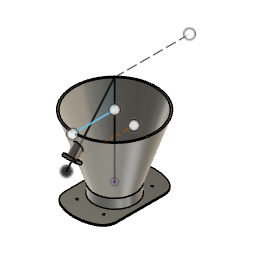
DroneVibrationSensorDeploymentCone-Remake v3 (Autodesk Fusion 360 design; units mm, degrees)
Autodesk Fusion 360 part; units mm, degrees
note: some values were not read from the file. Chosen so that the rebuilt part matches the saved one: which bodies a step acts on; which face or edge a step refers to; which pieces of a blend or face edit are solid.
sketch "Sketch1" plane through (0, 0, 0) normal (0, 1, 0) x (1, 0, 0)
  line L0 (0, 0) -> (32.2, 0)
  line L1 (0, 0) -> (0, -100)
  line L2 (0, -100) -> (65.7, -100)
  line L3 (65.7, -100) -> (32.2, 0)
  dimension "d1" = 32.2
  dimension "d2" = 100
  dimension "d3" = 65.7
  constraint coincident L0.start L1.start
  constraint horizontal L0
  constraint perpendicular L0 L1
  constraint perpendicular L1 L2
  measures "d1" distance of L0.start L0.end
  measures "d2" distance of L0.start L1.end
  measures "d3" distance of L1.end L2.end
revolve "Revolve1" add sketch "Sketch1" angle 360 about axis through (0, 0, 0) along (0, 0, 1) makes body 1
shell "Shell1" thickness 2.5 removed faces 1 at (2.2714, -9.9517, 100) on bodies 1
sketch "Sketch2" plane through (0, 0, 0) normal (0, 0, -1) x (1, 0, 0)
  circle A0 centre (0, 0) radius 32.2
  line L0 (-21, -21) -> (21, -21)
  line L1 (21, -21) -> (21, 21)
  line L2 (21, 21) -> (-21, 21)
  line L3 (-21, 21) -> (-21, -21)
  circle A1 centre (0, 0) radius 32.5
  dimension "d6" = 42
  dimension "d7" = 42
  constraint horizontal L0
  constraint vertical L1
  constraint horizontal L2
  constraint vertical L3
  constraint coincident A0.centre A1.centre
  measures "d6" distance of L0.start L0.end
  measures "d7" distance of L0.start L2.end
extrude "Extrude1" add sketch "Sketch2" along normal blind 22.5 contours A0 | L0 L1 L2 L3 | A1 bodies 1
extrude "Extrude2" cut sketch "Sketch2" against normal blind 10 contours L0 L1 L2 L3 bodies 1
extrude "Extrude3" cut sketch "Sketch2" along normal blind 16 contours L0 L1 L2 L3 bodies 1
sketch "Sketch5" plane through (0, 0, -16) normal (0, 0, 1) x (-1, 0, 0)
  line L0 (21, -21) -> (21, 21)
  line L1 (21, 21) -> (-21, 21)
  line L2 (-21, 21) -> (-21, -21)
  line L3 (-21, -21) -> (21, -21)
  circle A0 centre (17.5, -17.5) radius 1.5
  circle A1 centre (-17.5, -17.5) radius 1.5
  circle A2 centre (17.5, 17.5) radius 1.5
  circle A3 centre (-17.5, 17.5) radius 1.5
  line L4 (21, 21) -> (28.894, 21) construction
  line L5 (18.4952, 13.5139) -> (3.4952, 13.5139)
  line L6 (3.4952, 13.5139) -> (3.4952, -1.4861)
  line L7 (3.4952, -1.4861) -> (18.4952, -1.4861)
  line L8 (18.4952, -1.4861) -> (18.4952, 13.5139)
  dimension "d17" = 15
  dimension "d18" = 15
  constraint horizontal L4
  constraint coincident L0.end L1.start
  constraint horizontal L5
  constraint vertical L6
  constraint horizontal L7
  constraint vertical L8
  measures "d17" distance of L5.start L5.end
  measures "d18" distance of L5.start L7.end
extrude "Extrude4" cut sketch "Sketch5" against normal blind 1 contours A0 | A1 | A2 | A3 | L5 L6 L7 L8 bodies 1
extrude "Extrude5" cut 1 faces at (-1.1612, -8.4698, -22.5) along direction (0, 0, 1) blind 5.5 on bodies 1 bodies 1
sketch "Sketch6" plane through (0, 0, -17) normal (0, 0, -1) x (1, 0, 0)
  circle A0 centre (-17.5, -17.5) radius 1.5
  line L0 (-18.4952, 13.5139) -> (-3.4952, 13.5139)
  line L1 (-3.4952, 13.5139) -> (-3.4952, -1.4861)
  line L2 (-3.4952, -1.4861) -> (-18.4952, -1.4861)
  line L3 (-18.4952, -1.4861) -> (-18.4952, 13.5139)
  circle A1 centre (17.5, -17.5) radius 1.5
  circle A2 centre (-17.5, 17.5) radius 1.5
  circle A3 centre (17.5, 17.5) radius 1.5
  circle A4 centre (0, 0) radius 32.5
  line L4 (-18.4952, 13.5139) -> (-3.4952, 13.5139)
  line L5 (-3.4952, 13.5139) -> (-3.4952, -1.4861)
  line L6 (-3.4952, -1.4861) -> (-18.4952, -1.4861)
  line L7 (-18.4952, -1.4861) -> (-18.4952, 13.5139)
  circle A5 centre (-17.5, 17.5) radius 1.5
  circle A6 centre (17.5, 17.5) radius 1.5
  circle A7 centre (17.5, -17.5) radius 1.5
  circle A8 centre (-17.5, -17.5) radius 1.5
  circle A9 centre (0, 0) radius 65
  line L8 (0, 0) -> (44.414, 0) construction
  line L9 (0, 0) -> (44.414, 0) construction
  line L10 (0, 0) -> (44.414, 0) construction
  line L11 (0, 0) -> (44.414, 0) construction
  circle A10 centre (21.2606, -38.9947) radius 1.5
  circle A11 centre (-21.2606, -38.9947) radius 1.5
  circle A12 centre (-21.2606, 38.9947) radius 1.5
  circle A13 centre (21.2606, 38.9947) radius 1.5
  line L12 (0, 0) -> (65, 0)
  line L13 (0, 0) -> (0, 65)
  line L14 (0, -65) -> (0, 0)
  line L15 (0, 0) -> (-65, 0)
  dimension "d23" = 130
  dimension "d32" = 3
  dimension "d33" = 3
  dimension "d34" = 3
  dimension "d35" = 3
  constraint horizontal L4
  constraint vertical L5
  constraint horizontal L6
  constraint vertical L7
  constraint coincident L1.end L2.start
  constraint coincident L0.start L3.end
  constraint concentric A2 A5
  constraint concentric A3 A6
  constraint concentric A1 A7
  constraint concentric A0 A8
  constraint coincident A4.centre A9.centre
  constraint horizontal L8
  constraint horizontal L9
  constraint horizontal L10
  constraint horizontal L11
  constraint coincident A9 L12.end
  constraint parallel L9 L12
  constraint coincident A9 L13.end
  constraint perpendicular L10 L13
  constraint coincident A9 L14.start
  constraint perpendicular L12 L14
  constraint coincident A9 L15.end
  constraint perpendicular L5 L15
  measures "d23" diameter of A9
  measures "d32" diameter of A10
  measures "d33" diameter of A11
  measures "d34" diameter of A12
  measures "d35" diameter of A13
extrude "Extrude6" add sketch "Sketch6" against normal blind 2 contours A4 A9 L13 L15 | A4 A9 L14 L15 | A4 A9 L12 L13 | A4 A9 L12 L14 bodies 1
sketch "Sketch7" plane through (0, 0, -17) normal (0, 0, -1) x (1, 0, 0)
  circle A0 centre (0, 0) radius 65
  circle A1 centre (21.2606, 38.9947) radius 1.5
  circle A2 centre (-21.2606, 38.9947) radius 1.5
  circle A3 centre (21.2606, -38.9947) radius 1.5
  circle A4 centre (-21.2606, -38.9947) radius 1.5
  circle A5 centre (-17.5, -17.5) radius 1.5
  line L0 (-18.4952, 13.5139) -> (-3.4952, 13.5139)
  line L1 (-3.4952, 13.5139) -> (-3.4952, -1.4861)
  line L2 (-3.4952, -1.4861) -> (-18.4952, -1.4861)
  line L3 (-18.4952, -1.4861) -> (-18.4952, 13.5139)
  circle A6 centre (17.5, -17.5) radius 1.5
  circle A7 centre (-17.5, 17.5) radius 1.5
  circle A8 centre (17.5, 17.5) radius 1.5
  line L4 (0, 0) -> (41.407, 0)
  line L5 (0, 0) -> (-41.407, 0)
  line L6 (-41.407, 0) -> (-41.407, 50.1045)
  line L7 (-41.407, 0) -> (-41.407, -50.1045)
  line L8 (41.407, 0) -> (41.407, 50.1045)
  line L9 (41.407, 50.1045) -> (41.407, -50.1045)
  dimension "d38" = 41.407
  dimension "d39" = 41.407
  constraint coincident A0.centre L4.start
  constraint horizontal L4
  constraint parallel L4 L5
  constraint coincident A0 L6.end
  constraint perpendicular L5 L6
  constraint coincident A0 L7.end
  constraint perpendicular L5 L7
  constraint coincident A0 L8.end
  constraint perpendicular L4 L8
  constraint coincident A0 L9.end
  constraint perpendicular L4 L9
  measures "d38" distance of A0.centre L4.end
  measures "d39" distance of A0.centre L5.end
extrude "Extrude7" cut sketch "Sketch7" against normal blind 2 contours A0 L8 L9 | A0 L6 L7 bodies 1
fillet "Fillet1" radius 22.5 4 edges at (-41.407, -50.1045, -16) (41.407, -50.1045, -16) (41.407, 50.1045, -16) (-41.407, 50.1045, -16) on bodies 1
sketch "Sketch8" plane through (0, 0, 0) normal (0, 0, 1) x (1, 0, 0)
  line L0 (7.25, -37.9) -> (-7.25, -37.9)
  line L1 (7.25, -37.9) -> (-7.25, -37.9)
  line L2 (-7.25, -37.9) -> (-7.25, -52)
  line L3 (-7.25, -52) -> (7.25, -52)
  line L4 (7.25, -52) -> (7.25, -37.9)
  line L5 (7.25, -37.9) -> (9.25, -37.9) construction
  line L6 (-7.25, -52) -> (-5.25, -52) construction
  line L7 (8.6642, -36.4858) -> (-8.6642, -36.4858)
  line L8 (-8.6642, -36.4858) -> (-8.6642, -53.4142)
  line L9 (-8.6642, -53.4142) -> (8.6642, -53.4142)
  line L10 (8.6642, -53.4142) -> (8.6642, -36.4858)
  dimension "d47" = 14.5
  constraint horizontal L1
  constraint vertical L2
  constraint horizontal L3
  constraint vertical L4
  constraint horizontal L5
  constraint horizontal L6
  constraint horizontal L7
  constraint vertical L8
  constraint horizontal L9
  constraint vertical L10
  measures "d47" distance of L0.start L0.end
extrude "Extrude8" add sketch "Sketch8" along normal blind 3 separate body makes body 2
sketch "Sketch9" plane through (0, 0, 3) normal (0, 0, 1) x (-1, 0, 0)
  line L0 (-7.25, 37.9) -> (-7.25, 52)
  line L1 (-7.25, 52) -> (7.25, 52)
  line L2 (7.25, 52) -> (7.25, 37.9)
  line L3 (7.25, 37.9) -> (-7.25, 37.9)
  line L4 (-8.6642, 53.4142) -> (-8.6642, 36.4858)
  line L5 (-8.6642, 36.4858) -> (8.6642, 36.4858)
  line L6 (8.6642, 36.4858) -> (8.6642, 53.4142)
  line L7 (8.6642, 53.4142) -> (-8.6642, 53.4142)
  circle A0 centre (0, 45.5) radius 6
  circle A1 centre (0, 45.5) radius 7
  dimension "d54" = 12
  constraint concentric A0 A1
  measures "d54" diameter of A0
extrude "Extrude9" add sketch "Sketch9" along normal blind 1 contours L0 L1 L2 L3 A1 | L1 A1 | L1 A1 | L4 L5 L6 L7 bodies 2
sketch "Sketch10" plane through (0, 0, 4) normal (0, 0, 1) x (-1, 0, 0)
  circle A0 centre (0, 45.5) radius 6
  line L0 (8.6642, 53.4142) -> (-8.6642, 53.4142)
  line L1 (-8.6642, 53.4142) -> (-8.6642, 36.4858)
  line L2 (-8.6642, 36.4858) -> (8.6642, 36.4858)
  line L3 (8.6642, 36.4858) -> (8.6642, 53.4142)
  circle A1 centre (0, 45.5) radius 7
  dimension "d57" = 14
  constraint concentric A0 A1
  measures "d57" diameter of A1
move_body "Move1" bodies 2 to x (1, 0, 0) y (0, 0.866025, -0.5) z (0, 0.5, 0.866025) at (-4.0902, -14.8259, 8.0865)
sketch "Sketch11" plane through (4.574, 0, 0) normal (1, 0, 0) x (0, 1, 0)
  line L0 (-61.084, 34.7936) -> (-46.4235, 26.3294)
  line L1 (-46.4235, 26.3294) -> (-44.4235, 29.7935)
  line L2 (-44.4235, 29.7935) -> (-59.084, 38.2577)
  line L3 (-59.084, 38.2577) -> (-61.084, 34.7936)
  line L4 (-59.3519, 33.7936) -> (-58.3519, 35.5257)
  line L5 (-58.3519, 35.5257) -> (-54.8878, 33.5257)
  line L6 (-58.3519, 35.5257) -> (-54.3519, 35.5257) construction
  line L7 (-54.8878, 33.5257) -> (-55.8878, 31.7936)
  dimension "d65" = 2
  dimension "d66" = 30
  dimension "d67" = 4
  constraint perpendicular L2 L4
  constraint horizontal L6
  constraint coincident L0 L7.end
  constraint perpendicular L0 L7
  measures "d65" distance of L4.start L4.end
  measures "d66" angle of L5 L6
  measures "d67" distance of L4.end L5.end
extrude "Extrude13" cut sketch "Sketch11" against normal blind 2 contours L0 L4 L5 L7 bodies 2
move_body "Move2" bodies 2 to x (1, 0, 0) y (0, 1, 0) z (0, 0, 1) at (0, -11.0615, 32.5179)
move_body "Move3" bodies 2 to x (1, 0, 0) y (0, 1, 0) z (0, 0, 1) at (3.9246, -4.5574, 0)
sketch "Sketch13" plane through (0, 0, 0) normal (1, 0, 0) x (0, 1, 0)
  line L0 (0, 100) -> (-67.5, 100)
  line L1 (0, 0) -> (0, 145)
  line L2 (0, 145) -> (-77.1345, 53.0747)
  line L3 (0, 145) -> (120, 145) construction
  line L4 (-68.9683, 62.8068) -> (31.0317, 62.8068) construction
  dimension "d75" = 67.5
  dimension "d76" = 145
  dimension "d77" = 130
  dimension "d78" = 120
  constraint horizontal L0
  constraint coincident L1.start origin
  constraint vertical L1
  constraint horizontal L3
  constraint horizontal L4
  constraint coincident L2 L4.start
  measures "d75" distance of L0.start L0.end
  measures "d76" distance of L1.start L1.end
  measures "d77" angle of L2 L3
  measures "d78" distance of L1.end L2.end
move_body "Move4" bodies 2 to x (1, 0, 0) y (0, 0.984808, -0.173648) z (0, 0.173648, 0.984808) at (0, -11.891, -10.01)
sketch "Sketch14" plane through (0, 5.5476, 6.6114) normal (0, 0.642788, 0.766044) x (-1, 0, 0)
  circle A0 centre (0.1655, 94.843) radius 6
  line L0 (8.8298, 102.7572) -> (-8.4987, 102.7572)
  line L1 (-8.4987, 102.7572) -> (-8.4987, 85.8288)
  line L2 (-8.4987, 85.8288) -> (8.8298, 85.8288)
  line L3 (8.8298, 85.8288) -> (8.8298, 102.7572)
  circle A1 centre (0.1655, 94.843) radius 7
  dimension "d81" = 14
  constraint concentric A0 A1
  measures "d81" diameter of A1
extrude "Extrude16" cut sketch "Sketch14" along normal blind 25 contours A1 bodies 1 makes body 3 at (-20.0302, -57.4828, 85.5899)
extrude "Extrude17" add sketch "Sketch14" along normal blind 25 contours A1 bodies 1 2 3
delete_face "DeleteFace4" 1 faces at (-2.1561, -58.5907, 78.8965) on bodies 1
delete_face "DeleteFace5" 1 faces at (5.2275, -52.2324, 78.3586) on bodies 1
sketch "Sketch12" plane through (0, 1.7951, 3.1092) normal (0, 0.5, 0.866025) x (-1, 0, 0)
  circle A0 centre (4.0902, 62.3829) radius 6
  line L0 (12.7544, 70.2971) -> (-4.574, 70.2971)
  line L1 (-4.574, 70.2971) -> (-4.574, 53.3687)
  line L2 (-4.574, 53.3687) -> (12.7544, 53.3687)
  line L3 (12.7544, 53.3687) -> (12.7544, 70.2971)
  circle A1 centre (4.0902, 62.3829) radius 7
  dimension "d70" = 14
  constraint concentric A0 A1
  measures "d70" diameter of A1
extrude "Extrude14" [rolled back] along distance 25 taper angle 0
extrude "Extrude15" [rolled back] along distance 25 taper angle 0
delete_face "DeleteFace2" [rolled back]
delete_face "DeleteFace3" [rolled back]
